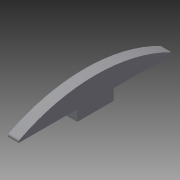
# Autodesk Inventor part: Camera Blinder 25090213
Saved by Autodesk Inventor 2013 (Build 170138000, 138)
## iProperties
Created: 2013-09-02
Part Number: Camera Blinder 25090213
Material: Generic
Document SubType Name: Modeling
Designer: Eric
Density: 1 g/cm^3
Author: Eric
Autodesk Inventor part; units mm, degrees
ref_plane "YZ Plane" through (0, 0, 0) normal (1, 0, 0) x (0, 1, 0)
ref_plane "XZ Plane" through (0, 0, 0) normal (0, 1, 0) x (-1, 0, 0)
ref_plane "XY Plane" through (0, 0, 0) normal (0, 0, 1) x (1, 0, 0)
sketch "Sketch1" plane through (0, 0, 0) normal (1, 0, 0) x (0, 1, 0)
  line L0 (-5, 40.398) -> (-5, 37.398)
  line L1 (-5, 37.398) -> (5, 37.398)
  line L2 (5, 37.398) -> (5, 40.398)
  line L3 (-21, 40.398) -> (-5, 40.398)
  line L4 (5, 40.398) -> (21, 40.398)
  line L5 (-21, 40.398) -> (-21, 40.6202)
  line L6 (21, 40.398) -> (21, 40.6202)
  arc A0 (-20.7253, 41.0666) -> (-21, 40.6202) centre (-20.5, 40.6202) ccw
  arc A1 (21, 40.6202) -> (20.7253, 41.0666) centre (20.5, 40.6202) ccw
  arc A2 (20.7253, 41.0666) -> (-20.7253, 41.0666) centre (0, 0) ccw
  point P0 (0, 37.398)
  dimension "d3" = 10
  dimension "d6" = 3
  dimension "d7" = 42
  dimension "d8" = 16
  dimension "d9" = 0.5
  dimension "d10" = 37.398
  constraints: 14 end point, 7 perpendicular, 6 point on circle, 3 centre point, 2 horizontal, 2 tangent, 1 coincident, 1 collinear, 1 equal radius, 1 midpoint, 1 vertical alignment
  measures "d3" distance of L0.end L1.end
  measures "d6" distance between parallel lines of L1 L3
  measures "d7" distance between parallel lines of L6 L5
  measures "d8" distance between parallel lines of L0 L5
  measures "d9" radius of A0
  measures "d10" distance from line of point (0, 0) L1
extrude "Extrusion1" add sketch "Sketch1" along normal blind 3
body "Solid1"
